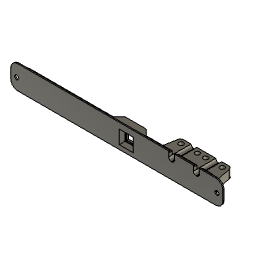
CoverWithCables (Autodesk Fusion 360 design; units mm, degrees)
Autodesk Fusion 360 part; units mm, degrees
note: some values were not read from the file. Chosen so that the rebuilt part matches the saved one: which face or edge a step refers to.
sketch "Skizze1" plane through (0, 0, 0) normal (0, 1, 0) x (1, 0, 0)
  line L0 (0, 0) -> (164, 0)
  line L1 (164, 0) -> (164, -18)
  line L2 (164, -18) -> (0, -18)
  line L3 (0, -18) -> (0, 0)
  dimension "d1" = 18
  dimension "d2" = 164
  constraint horizontal L0
  constraint vertical L1
  constraint horizontal L2
  constraint vertical L3
  constraint coincident L0.start L3.end
  measures "d1" distance of L0.start L2.end
  measures "d2" distance of L1.end L2.end
extrude "Extrusion1" add sketch "Skizze1" along normal blind 8 makes body 1
fillet "Abrundung1" radius 5 4 edges at (0, 4, 18) (164, 4, 18) (0, 4, 0) (164, 4, 0) on bodies 1
sketch "Skizze2" plane through (0, 0, 0) normal (0, 1, 0) x (1, 0, 0)
  line L0 (-8, -19.5) -> (172, -19.5)
  line L1 (172, -19.5) -> (172, 0.5)
  line L2 (172, 0.5) -> (-8, 0.5)
  line L3 (-8, 0.5) -> (-8, -19.5)
  line L4 (-8, -9) -> (172, -9) construction
  circle A0 centre (-3, -9) radius 1.75
  circle A1 centre (167, -9) radius 1.75
  point P0 (0, -13)
  point P1 (164, -13)
  dimension "d7" = 0.5
  dimension "d8" = 19.5
  dimension "d9" = 9
  dimension "d10" = 3
  dimension "d11" = 3
  dimension "d12" = 3.5
  dimension "d13" = 5
  dimension "d14" = 5
  constraint horizontal L0
  constraint vertical L1
  constraint horizontal L2
  constraint vertical L3
  constraint coincident L3 L4.start
  constraint coincident L1 L4.end
  constraint perpendicular L1 L4
  constraint coincident L4 A0.centre
  constraint coincident L4 A1.centre
  constraint equal A0 A1
  measures "d7" vertical distance of origin L2.end
  measures "d8" vertical distance of origin L0.start
  measures "d9" vertical distance of origin L4.start
  measures "d10" horizontal distance of A0.centre P0
  measures "d11" horizontal distance of A1.centre P1
  measures "d12" diameter of A0
  measures "d13" horizontal distance of L0.start A0.centre
  measures "d14" distance of L4.end A1.centre
extrude "Extrusion2" add sketch "Skizze2" against normal blind 1 bodies 1
fillet "Abrundung2" radius 6 4 edges at (172, -0.5, 19.5) (172, -0.5, -0.5) (-8, -0.5, 19.5) (-8, -0.5, -0.5) on bodies 1
extrude "Extrusion3" cut 1 faces at (56.3333, 8, 12) along direction (0, -1, 0) blind 6 on bodies 1 bodies 1
sketch "Skizze3" plane through (0, 2, 0) normal (0, 1, 0) x (-1, 0, 0)
  arc A0 (-164, 5) -> (-159, 0) centre (-159, 5) ccw
  line L0 (-159, 0) -> (-5, 0)
  arc A1 (-5, 0) -> (0, 5) centre (-5, 5) ccw
  line L1 (0, 5) -> (0, 13)
  arc A2 (0, 13) -> (-5, 18) centre (-5, 13) ccw
  line L2 (-5, 18) -> (-159, 18)
  arc A3 (-159, 18) -> (-164, 13) centre (-159, 13) ccw
  line L3 (-164, 13) -> (-164, 5)
  line L4 (-96, 14.5) -> (-84, 14.5)
  line L5 (-84, 14.5) -> (-84, 3)
  line L6 (-84, 3) -> (-96, 3)
  line L7 (-96, 3) -> (-96, 14.5)
  dimension "d21" = 68
  dimension "d22" = 3
  dimension "d23" = 3.5
  dimension "d24" = 12
  constraint horizontal L4
  constraint vertical L5
  constraint horizontal L6
  constraint vertical L7
  measures "d21" horizontal distance of A3.end L4.start
  measures "d22" vertical distance of A0.end L6.end
  measures "d23" vertical distance of L2.end L4.start
  measures "d24" distance of L4.start L4.end
extrude "Extrusion4" add sketch "Skizze3" along normal blind 3 contours L4 L5 L6 L7 bodies 1
sketch "Skizze4" plane through (0, 2, 0) normal (0, 1, 0) x (-1, 0, 0)
  line L0 (-96, 3) -> (-96, 14.5)
  line L1 (-96, 14.5) -> (-84, 14.5)
  line L2 (-84, 14.5) -> (-84, 3)
  line L3 (-84, 3) -> (-96, 3)
  arc A0 (-164, 5) -> (-159, 0) centre (-159, 5) ccw
  line L4 (-159, 0) -> (-5, 0)
  arc A1 (-5, 0) -> (0, 5) centre (-5, 5) ccw
  line L5 (0, 5) -> (0, 13)
  arc A2 (0, 13) -> (-5, 18) centre (-5, 13) ccw
  line L6 (-5, 18) -> (-159, 18)
  arc A3 (-159, 18) -> (-164, 13) centre (-159, 13) ccw
  line L7 (-164, 13) -> (-164, 5)
  line L8 (-99, 18) -> (-81, 18)
  line L9 (-81, 18) -> (-81, 0)
  line L10 (-81, 0) -> (-99, 0)
  line L11 (-99, 0) -> (-99, 18)
  dimension "d27" = 3.5
  dimension "d28" = 3
  dimension "d29" = 3
  dimension "d30" = 3
  constraint horizontal L8
  constraint vertical L9
  constraint horizontal L10
  constraint vertical L11
  measures "d27" vertical distance of L0.end L8.start
  measures "d28" vertical distance of L0.start L10.end
  measures "d29" horizontal distance of L0.end L8.start
  measures "d30" horizontal distance of L1.end L8.end
extrude "Extrusion5" add sketch "Skizze4" along normal blind 5 contours L4 L6 L8 L9 L10 L11 bodies 1
sketch "Skizze5" plane through (0, 5, 0) normal (0, 1, 0) x (-1, 0, 0)
  line L0 (-96, 3) -> (-84, 3)
  line L1 (-84, 3) -> (-84, 14.5)
  line L2 (-84, 14.5) -> (-96, 14.5)
  line L3 (-96, 14.5) -> (-96, 3)
  line L4 (-95.5, 14) -> (-84.5, 14)
  line L5 (-84.5, 14) -> (-84.5, 3.5)
  line L6 (-84.5, 3.5) -> (-95.5, 3.5)
  line L7 (-95.5, 3.5) -> (-95.5, 14)
  dimension "d33" = 0.5
  dimension "d34" = 0.5
  dimension "d35" = 0.5
  dimension "d36" = 0.5
  constraint horizontal L4
  constraint vertical L5
  constraint horizontal L6
  constraint vertical L7
  measures "d33" vertical distance of L2.end L4.start
  measures "d34" horizontal distance of L1.end L4.end
  measures "d35" horizontal distance of L2.end L4.start
  measures "d36" vertical distance of L0.start L6.end
extrude "Extrusion6" cut sketch "Skizze5" against normal blind 13 contours L4 L5 L6 L7 bodies 1
sketch "Skizze6" plane through (0, -1, 0) normal (0, -1, 0) x (1, 0, 0)
  line L0 (84.5, 3.5) -> (84.5, 14)
  line L1 (84.5, 14) -> (95.5, 14)
  line L2 (95.5, 14) -> (95.5, 3.5)
  line L3 (95.5, 3.5) -> (84.5, 3.5)
  arc A0 (-8, 5.5) -> (-2, -0.5) centre (-2, 5.5) ccw
  line L4 (-2, -0.5) -> (166, -0.5)
  arc A1 (166, -0.5) -> (172, 5.5) centre (166, 5.5) ccw
  line L5 (172, 5.5) -> (172, 13.5)
  arc A2 (172, 13.5) -> (166, 19.5) centre (166, 13.5) ccw
  line L6 (166, 19.5) -> (-2, 19.5)
  arc A3 (-2, 19.5) -> (-8, 13.5) centre (-2, 13.5) ccw
  line L7 (-8, 13.5) -> (-8, 5.5)
  circle A4 centre (-3, 9) radius 1.75
  circle A5 centre (167, 9) radius 1.75
  line L8 (84, 14.5) -> (96, 14.5)
  line L9 (96, 14.5) -> (96, 3)
  line L10 (96, 3) -> (84, 3)
  line L11 (84, 3) -> (84, 14.5)
  dimension "d39" = 0.5
  dimension "d40" = 0.5
  dimension "d41" = 0.5
  dimension "d42" = 0.5
  constraint horizontal L8
  constraint vertical L9
  constraint horizontal L10
  constraint vertical L11
  measures "d39" horizontal distance of L0.end L8.start
  measures "d40" horizontal distance of L1.end L8.end
  measures "d41" vertical distance of L2.end L9.end
  measures "d42" vertical distance of L0.end L8.start
extrude "Extrusion7" cut sketch "Skizze6" against normal blind 5 contours L8 L9 L10 L11 bodies 1
sketch "Skizze7" plane through (0, 2, 0) normal (0, 1, 0) x (-1, 0, 0)
  line L0 (-99, 0) -> (-99, 18)
  line L1 (-99, 18) -> (-159, 18)
  arc A0 (-159, 18) -> (-164, 13) centre (-159, 13) ccw
  line L2 (-164, 13) -> (-164, 5)
  arc A1 (-164, 5) -> (-159, 0) centre (-159, 5) ccw
  line L3 (-159, 0) -> (-99, 0)
  line L4 (-152, 18) -> (-152, 15)
  line L5 (-147, 18) -> (-147, 15)
  line L6 (-149.75, 12.75) -> (-149.25, 12.75)
  arc A2 (-152, 15) -> (-149.75, 12.75) centre (-149.75, 15) ccw
  arc A3 (-149.25, 12.75) -> (-147, 15) centre (-149.25, 15) ccw
  line L7 (-131, 18) -> (-131, 15)
  line L8 (-128.75, 12.75) -> (-128.25, 12.75)
  line L9 (-126, 15) -> (-126, 18)
  arc A4 (-131, 15) -> (-128.75, 12.75) centre (-128.75, 15) ccw
  arc A5 (-128.25, 12.75) -> (-126, 15) centre (-128.25, 15) ccw
  dimension "d46" = 2.25
  dimension "d47" = 2.25
  dimension "d49" = 5
  dimension "d50" = 3
  dimension "d51" = 2.25
  dimension "d52" = 2.25
  dimension "d53" = 5
  dimension "d54" = 16
  dimension "d55" = 7
  dimension "d56" = 3
  constraint coincident L1 L4.start
  constraint perpendicular L1 L4
  constraint coincident L1 L5.start
  constraint perpendicular L1 L5
  constraint perpendicular L5 L6
  constraint tangent L4 A2
  constraint tangent L6 A2
  constraint tangent L5 A3
  constraint tangent L6 A3
  constraint coincident L1 L7.start
  constraint perpendicular L1 L7
  constraint perpendicular L7 L8
  constraint coincident L1 L9.end
  constraint perpendicular L1 L9
  constraint tangent L7 A4
  constraint tangent L8 A4
  constraint tangent L8 A5
  constraint tangent L9 A5
  measures "d46" radius of A2
  measures "d47" radius of A3
  measures "d49" distance of L4.start L5.start
  measures "d50" distance of L5.start L5.end
  measures "d51" radius of A4
  measures "d52" radius of A5
  measures "d53" distance of L7.start L9.end
  measures "d54" distance of L5.start L7.start
  measures "d55" distance of L1.end L4.start
  measures "d56" distance of L7.start L7.end
extrude "Extrusion8" cut sketch "Skizze7" against normal blind 6 contours L1 L7 L8 L9 A4 A5 | L1 L4 L5 L6 A2 A3 bodies 1
extrude "Extrusion9" cut 2 faces at (148.6667, -0.3333, 18) (127.6667, -0.3333, 18) along direction (0, 0, 1) blind 3 on bodies 1 bodies 1
sketch "Skizze8" plane through (0, 2, 0) normal (0, 1, 0) x (-1, 0, 0)
  line L0 (-147, 18) -> (-147, 15)
  arc A0 (-149.25, 12.75) -> (-147, 15) centre (-149.25, 15) ccw
  line L1 (-149.25, 12.75) -> (-149.75, 12.75)
  arc A1 (-152, 15) -> (-149.75, 12.75) centre (-149.75, 15) ccw
  line L2 (-152, 15) -> (-152, 18)
  line L3 (-152, 18) -> (-159, 18)
  arc A2 (-159, 18) -> (-164, 13) centre (-159, 13) ccw
  line L4 (-164, 13) -> (-164, 5)
  arc A3 (-164, 5) -> (-159, 0) centre (-159, 5) ccw
  line L5 (-159, 0) -> (-99, 0)
  line L6 (-99, 0) -> (-99, 18)
  line L7 (-99, 18) -> (-126, 18)
  line L8 (-126, 18) -> (-126, 15)
  arc A4 (-128.25, 12.75) -> (-126, 15) centre (-128.25, 15) ccw
  line L9 (-128.25, 12.75) -> (-128.75, 12.75)
  arc A5 (-131, 15) -> (-128.75, 12.75) centre (-128.75, 15) ccw
  line L10 (-131, 15) -> (-131, 18)
  line L11 (-131, 18) -> (-147, 18)
  line L12 (-152, 15) -> (-160.5, 15)
  line L13 (-160.5, 15) -> (-160.5, 8)
  line L14 (-160.5, 8) -> (-117.5, 8)
  line L15 (-117.5, 8) -> (-117.5, 15)
  line L16 (-117.5, 15) -> (-126, 15)
  line L17 (-147, 15) -> (-131, 15)
  dimension "d61" = 3
  dimension "d62" = 3
  dimension "d63" = 8.5
  dimension "d64" = 7
  dimension "d65" = 8.5
  constraint coincident L2 A1.start
  constraint perpendicular L2 L12
  constraint perpendicular L12 L13
  constraint perpendicular L2 L14
  constraint perpendicular L14 L15
  constraint coincident L8 A4.end
  constraint perpendicular L8 L16
  constraint coincident L0.end A0.end
  constraint coincident A5.start L10.start
  measures "d61" distance of L2.end A1.start
  measures "d62" distance of L7.end L8.end
  measures "d63" distance of A1.start L12.end
  measures "d64" distance of L12.end L13.end
  measures "d65" distance of L15.end L8.end
extrude "Extrusion10" add sketch "Skizze8" along normal blind 16 contours A0 L1 A1 A4 L9 A5 L12 L13 L14 L15 L16 L17 bodies 1
hole "Bohrung1" at (156.5, 14, 15) direction (0, 0, -1) diameter 4 depth 7 tip angle 180 bodies 1
hole "Bohrung2" at (142.5, 14, 15) direction (0, 0, -1) diameter 4 depth 7 tip angle 180 bodies 1
hole "Bohrung3" at (135.5, 14, 15) direction (0, 0, -1) diameter 4 depth 7 tip angle 180 bodies 1
hole "Bohrung4" at (121.5, 14, 15) direction (0, 0, -1) diameter 4 depth 7 tip angle 180 bodies 1
chamfer "Fase1" distance 5 angle 45 2 edges at (99, 2, 9) (81, 2, 9) on bodies 1
chamfer "Fase2" distance 3 distance2 16 2 edges at (160.5, 2, 11.5) (117.5, 2, 11.5) measured on face at (108.4993, 2, 8.6667) measured on face at (108.4993, 2, 8.6667) on bodies 1
sketch "Skizze10" plane through (0, 0, 0) normal (0, 1, 0) x (1, 0, 0)
  line L0 (160, -15.25) -> (152, -15.25)
  line L1 (152, -15.25) -> (152, -15.338)
  line L2 (150, -17.338) -> (149, -17.338)
  line L3 (147, -15.338) -> (147, -15.25)
  line L4 (147, -15.25) -> (139, -15.25)
  line L5 (139, -15.25) -> (139, -16.75)
  line L6 (139, -16.75) -> (145.5, -16.75)
  line L7 (145.5, -16.75) -> (145.7518, -17.2759)
  line L8 (148.2321, -18.838) -> (150.7679, -18.838)
  line L9 (153.2482, -17.2759) -> (153.5, -16.75)
  line L10 (153.5, -16.75) -> (160, -16.75)
  line L11 (160, -16.75) -> (160, -15.25)
  arc A0 (150, -17.338) -> (152, -15.338) centre (150, -15.338) ccw
  arc A1 (147, -15.338) -> (149, -17.338) centre (149, -15.338) ccw
  arc A2 (145.7518, -17.2759) -> (148.2321, -18.838) centre (148.2321, -16.088) ccw
  arc A3 (150.7679, -18.838) -> (153.2482, -17.2759) centre (150.7679, -16.088) ccw
  point P0 (146.5, -18.838)
  point P1 (152.5, -18.838)
  point P2 (147, -19.5)
  point P3 (152, -19.5)
  point P4 (152, -18)
  point P5 (147, -18)
  dimension "d97" = 5
  dimension "d98" = 5
  dimension "d99" = 2
  dimension "d100" = 2
  dimension "d101" = 1.5
  dimension "d102" = 1.5
  dimension "d103" = 8
  dimension "d104" = 8
  dimension "d105" = 1.5
  dimension "d106" = 1.5
  dimension "d107" = 1
  dimension "d108" = 1
  dimension "d109" = 2.75
  dimension "d110" = 2.75
  dimension "d112" = 1.5
  dimension "d113" = 2.75
  dimension "d114" = 2.75
  constraint horizontal L0
  constraint perpendicular L0 L1
  constraint perpendicular L1 L2
  constraint perpendicular L2 L3
  constraint perpendicular L3 L4
  constraint perpendicular L4 L5
  constraint parallel L4 L8
  constraint parallel L4 L10
  constraint vertical L11
  constraint tangent L1 A0
  constraint tangent L2 A0
  constraint tangent L2 A1
  constraint tangent L3 A1
  constraint horizontal L6
  constraint coincident P0 L7
  constraint coincident P0 L8
  constraint tangent L7 A2
  constraint tangent L8 A2
  constraint coincident P1 L8
  constraint coincident P1 L9
  constraint tangent L8 A3
  constraint tangent L9 A3
  measures "d97" horizontal distance of L0.end P2
  measures "d98" horizontal distance of L3.end P3
  measures "d99" radius of A0
  measures "d100" radius of A1
  measures "d101" horizontal distance of L0.end L9.end
  measures "d102" distance of L0.start L10.end
  measures "d103" distance of L0.start L0.end
  measures "d104" distance of L3.end L4.end
  measures "d105" distance of L4.end L5.end
  measures "d106" horizontal distance of L6.end L3.start
  measures "d107" horizontal distance of L6.end P0
  measures "d108" horizontal distance of P1 L9.end
  measures "d109" radius of A2
  measures "d110" radius of A3
  measures "d112" vertical distance of L2.start L8.end
  measures "d113" distance of L0.end P4
  measures "d114" distance of L3.end P5
extrude "Extrusion11" add sketch "Skizze10" along normal blind 8 separate body makes body 2
move_body "Verschieben1" bodies 1 to x (1, 0, 0) y (0, 1, 0) z (0, 0, 1) at (0, -8, 0)
move_body "Verschieben2" bodies 2 to x (1, 0, 0) y (0, 1, 0) z (0, 0, 1) at (0, 1, 0)
hole "Bohrung5" at (142.5, 5, 16.75) direction (0, 0, -1) diameter 3.2 depth 7 tip angle 180 bodies 2
hole "Bohrung6" at (156.5, 5, 16.75) direction (0, 0, -1) diameter 3.2 depth 7 tip angle 180 bodies 2
move_body "Verschieben3" bodies 2 to x (1, 0, 0) y (0, 1, 0) z (0, 0, 1) at (0, 1, 0)
fillet "Abrundung6" radius 3 4 edges at (160, 10, 16) (160, 2, 16) (139, 10, 16) (139, 2, 16) on bodies 2
fillet "Abrundung7" radius 3 8 edges at (160.5, 9.9984, 15) (160.5, 9.9968, 11.5) (160.5, 9.9984, 8) (117.5, 9.9984, 8) (117.5, 9.9968, 11.5) (117.5, 9.9984, 15) (160.5, 10, 11.5) (117.5, 10, 11.5) on bodies 1
hidden bodies 2
